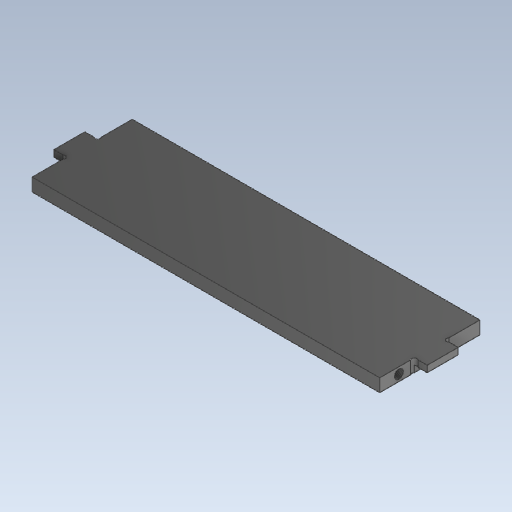
# Autodesk Inventor part: Cockpit_battery_bottom_frame
Saved by Autodesk Inventor 2020 (Build 240168000, 168)
## iProperties
Created: 2022-04-24
Part Number: Cockpit_battery_bottom_frame
Material: アセタール樹脂、黒
Document SubType Name: Modeling
Designer: Masato Kubotera
Density: 1.425 g/cm^3
Appearance: 滑らか - 黒
Description: POM T5
Author: Masato Kubotera
Autodesk Inventor part; units mm, degrees
ref_plane "YZ Plane" through (0, 0, 0) normal (1, 0, 0) x (0, 1, 0)
ref_plane "XZ Plane" through (0, 0, 0) normal (0, 1, 0) x (-1, 0, 0)
derived "Cockpit_side_frame.ipt"
sketch "スケッチ2" plane through (0, 0, 0) normal (0, 1, 0) x (-1, 0, 0)
  line L0 (-23.5, -22.5) -> (-28.5, -27.5)
  line L1 (-28.5, -27.5) -> (-28.5, -91)
  line L2 (-28.5, -91) -> (-23.5, -96)
  line L3 (-23.5, -96) -> (35.75, -96)
  line L4 (37.75, -98) -> (37.75, -131)
  line L5 (37.75, -131) -> (42.75, -136)
  line L6 (42.75, -136) -> (83.5, -136)
  line L7 (88.5, -131) -> (88.5, -20)
  line L8 (88.5, -20) -> (86, -17.5)
  line L9 (86, -17.5) -> (80.25, -17.5)
  line L10 (80.25, -17.5) -> (80.25, -22.5)
  line L11 (80.25, -22.5) -> (73.9849, -22.5)
  line L12 (72.5, -21.0151) -> (72.5, -17.5)
  line L13 (72.5, -17.5) -> (64.5, -17.5)
  line L14 (64.5, -17.5) -> (64.5, -21.0151)
  line L15 (63.0151, -22.5) -> (-23.5, -22.5)
  line L16 (-25.25, -25) -> (-20.25, -25) construction
  line L17 (-20.25, -25) -> (-20.25, -93.5) construction
  line L18 (-20.25, -93.5) -> (-25.25, -93.5) construction
  line L19 (-25.25, -93.5) -> (-25.25, -25) construction
  line L20 (-26, -25) -> (-25.25, -25) construction
  line L21 (-25.25, -93.5) -> (-26, -93.5) construction
  line L22 (-26, -93.5) -> (-26, -25) construction
  line L23 (-20.25, -93.5) -> (80.25, -93.5) construction
  line L24 (-20.25, -88.5) -> (80.25, -88.5) construction
  line L25 (80.25, -22.5) -> (80.25, -90.5) construction
  line L26 (80.25, -90.5) -> (85.25, -90.5) construction
  line L27 (85.25, -90.5) -> (85.25, -22.5) construction
  line L28 (80.25, -88.5) -> (80.25, -93.5) construction
  line L29 (80.25, -91) -> (85.25, -91) construction
  line L30 (85.25, -91) -> (85.25, -133.5) construction
  line L31 (80.25, -91) -> (80.25, -133.5) construction
  line L32 (80.25, -133.5) -> (85.25, -133.5) construction
  line L33 (40.25, -133.5) -> (40.25, -128.5) construction
  line L34 (40.25, -128.5) -> (40.25, -93.5) construction
  line L35 (45.25, -93.5) -> (45.25, -128.5) construction
  line L36 (40.25, -128.5) -> (45.25, -128.5) construction
  line L37 (42.75, -128.5) -> (42.75, -93.5) construction
  line L38 (40.25, -128.5) -> (79.1145, -128.5) construction
  line L39 (79.1145, -128.5) -> (79.1145, -133.5) construction
  line L40 (79.1145, -133.5) -> (40.25, -133.5) construction
  line L41 (40.25, -131) -> (79.1145, -131) construction
  line L42 (82.75, -91) -> (82.75, -133.5) construction
  circle A0 centre (82.75, -131) radius 2
  arc A1 (80.25, -128.5) -> (85.25, -128.5) centre (82.75, -131) ccw construction
  line L43 (80.25, -91) -> (-20.25, -91) construction
  line L44 (42.75, -111) -> (45.25, -111) construction
  line L45 (59.6822, -128.5) -> (59.6822, -131) construction
  line L46 (42.7, -115.5651) -> (42.7, -106.4349)
  line L47 (45.3, -107.05) -> (45.3, -114.95)
  line L48 (45.3, -117.05) -> (42.7, -104.95) construction
  line L49 (42.7, -117.05) -> (45.3, -104.95) construction
  line L50 (55.7322, -128.45) -> (63.6322, -128.45)
  line L51 (64.2473, -131.05) -> (55.1172, -131.05)
  line L52 (53.6322, -128.45) -> (65.7322, -131.05) construction
  line L53 (65.7322, -128.45) -> (53.6322, -131.05) construction
  line L54 (42.75, -105) -> (45.25, -105) construction
  line L55 (42.75, -117) -> (45.25, -117) construction
  arc A2 (44.1849, -104.95) -> (42.7, -106.4349) centre (43.4425, -105.6925) ccw
  arc A3 (45.3, -107.05) -> (45.3, -104.95) centre (45.3, -106) ccw
  arc A4 (42.7, -115.5651) -> (44.1849, -117.05) centre (43.4425, -116.3075) ccw
  arc A5 (45.3, -117.05) -> (45.3, -114.95) centre (45.3, -116) ccw
  line L56 (53.6822, -131) -> (53.6822, -128.5) construction
  line L57 (65.6822, -128.5) -> (65.6822, -131) construction
  arc A6 (53.6322, -129.5651) -> (55.1172, -131.05) centre (54.3747, -130.3075) ccw
  arc A7 (55.7322, -128.45) -> (53.6322, -128.45) centre (54.6822, -128.45) ccw
  arc A8 (64.2473, -131.05) -> (65.7322, -129.5651) centre (64.9898, -130.3075) ccw
  arc A9 (65.7322, -128.45) -> (63.6322, -128.45) centre (64.6822, -128.45) ccw
  line L58 (53.6322, -129.5651) -> (53.6322, -128.45)
  line L59 (65.7322, -128.45) -> (65.7322, -129.5651)
  line L60 (44.1849, -104.95) -> (45.3, -104.95)
  line L61 (45.3, -117.05) -> (44.1849, -117.05)
  circle A10 centre (47.6822, -131) radius 1.6
  line L62 (85.25, -22.5) -> (85.25, -17.5) construction
  line L63 (86, -17.5) -> (86, -90.5) construction
  line L64 (86, -90.5) -> (85.25, -90.5) construction
  line L65 (-18.5, -82.5) -> (-18.5, -61)
  arc A11 (-18.5, -82.5) -> (-16.5, -84.5) centre (-16.5, -82.5) ccw
  line L66 (45.5, -84.5) -> (-16.5, -84.5)
  arc A12 (45.5, -84.5) -> (47.5, -82.5) centre (45.5, -82.5) ccw
  line L67 (47.5, -61) -> (47.5, -82.5)
  arc A13 (47.5, -61) -> (45.5, -59) centre (45.5, -61) ccw
  line L68 (-16.5, -59) -> (45.5, -59)
  arc A14 (-16.5, -59) -> (-18.5, -61) centre (-16.5, -61) ccw
  line L69 (30, -88.5) -> (30, -91) construction
  line L70 (82.75, -22.5) -> (82.75, -90.5) construction
  circle A15 centre (82.75, -34) radius 1.6
  circle A16 centre (82.75, -34) radius 3
  circle A17 centre (82.75, -79) radius 3
  circle A18 centre (82.75, -79) radius 1.6
  line L71 (85.25, -22.5) -> (80.25, -22.5) construction
  arc A19 (85.25, -91) -> (80.25, -91) centre (82.75, -131) ccw construction
  circle A20 centre (47.6822, -131) radius 3
  circle A21 centre (42.75, -99) radius 1.6
  circle A22 centre (42.75, -99) radius 3
  line L72 (5, -88.5) -> (5, -91) construction
  line L73 (55, -88.5) -> (55, -91) construction
  line L74 (53.5651, -91.05) -> (6.4349, -91.05)
  line L75 (4.95, -89.5651) -> (4.95, -88.45)
  line L76 (7.05, -88.45) -> (52.95, -88.45)
  line L77 (55.05, -88.45) -> (55.05, -89.5651)
  line L78 (55.05, -91.05) -> (4.95, -88.45) construction
  line L79 (4.95, -91.05) -> (55.05, -88.45) construction
  arc A23 (7.05, -88.45) -> (4.95, -88.45) centre (6, -88.45) ccw
  arc A24 (4.95, -89.5651) -> (6.4349, -91.05) centre (5.6925, -90.3075) ccw
  arc A25 (53.5651, -91.05) -> (55.05, -89.5651) centre (54.3075, -90.3075) ccw
  arc A26 (55.05, -88.45) -> (52.95, -88.45) centre (54, -88.45) ccw
  line L80 (-20.25, -41) -> (80.25, -41) construction
  line L81 (80.25, -36) -> (-20.25, -36) construction
  line L82 (-20.25, -36) -> (-20.25, -41) construction
  line L83 (-20.25, -38.5) -> (80.25, -38.5) construction
  line L84 (30, -41) -> (30, -36) construction
  line L85 (53.5651, -35.95) -> (6.4349, -35.95)
  line L86 (6.4349, -41.05) -> (53.5651, -41.05)
  line L87 (55.05, -35.95) -> (4.95, -41.05) construction
  line L88 (4.95, -35.95) -> (55.5723, -41.1032) construction
  arc A27 (6.4349, -35.95) -> (4.95, -37.4349) centre (5.6925, -36.6925) ccw
  arc A28 (4.95, -39.5651) -> (6.4349, -41.05) centre (5.6925, -40.3075) ccw
  arc A29 (55.05, -37.4349) -> (53.5651, -35.95) centre (54.3075, -36.6925) ccw
  arc A30 (53.5651, -41.05) -> (55.05, -39.5651) centre (54.3075, -40.3075) ccw
  line L89 (5, -41) -> (5, -36) construction
  line L90 (55, -36) -> (55, -41) construction
  line L91 (4.95, -37.4349) -> (4.95, -39.5651)
  line L92 (55.05, -39.5651) -> (55.05, -37.4349)
  circle A31 centre (-2.5, -38.5) radius 1.6
  circle A32 centre (-2.5, -38.5) radius 3
  circle A33 centre (62.5, -38.5) radius 1.6
  circle A34 centre (62.5, -38.5) radius 3
  line L93 (-25.25, -44.25) -> (-22.75, -44.25) construction
  line L94 (-25.25, -49.25) -> (-26, -49.25) construction
  line L95 (-25.25, -74.25) -> (-22.75, -74.25) construction
  line L96 (-25.25, -69.25) -> (-26, -69.25) construction
  line L97 (-26, -59.25) -> (-25.25, -59.25) construction
  line L98 (-25.25, -59.25) -> (-22.75, -59.25) construction
  line L99 (-22.75, -25) -> (-22.75, -93.5) construction
  arc A35 (63.0151, -22.5) -> (64.5, -21.0151) centre (63.7575, -21.7575) ccw
  arc A36 (72.5, -21.0151) -> (73.9849, -22.5) centre (73.2425, -21.7575) ccw
  line L100 (56.75, -22.5) -> (56.75, -32.5) construction
  line L101 (56.75, -32.5) -> (80.25, -32.5) construction
  line L102 (80.25, -32.5) -> (80.25, -22.5) construction
  line L103 (68.5, -17.5) -> (68.5, -32.5) construction
  line L104 (60.5, -22.5) -> (60.5, -17.5) construction
  line L105 (76.5, -22.5) -> (76.5, -17.5) construction
  line L106 (-22.7, -46.3) -> (-22.7, -72.2)
  line L107 (-25.3, -72.8151) -> (-25.3, -69.564)
  line L108 (-25.3, -44.2) -> (-22.7, -74.3) construction
  line L109 (-22.7, -44.2) -> (-25.3, -74.3) construction
  arc A37 (-22.7, -46.3) -> (-22.7, -44.2) centre (-22.7, -45.25) ccw
  arc A38 (-23.8151, -44.2) -> (-25.3, -45.6849) centre (-24.5575, -44.9425) ccw
  line L110 (-23.8151, -44.2) -> (-22.7, -44.2)
  arc A39 (-25.3, -72.8151) -> (-23.8151, -74.3) centre (-24.5575, -73.5575) ccw
  arc A40 (-22.7, -74.3) -> (-22.7, -72.2) centre (-22.7, -73.25) ccw
  line L111 (-22.7, -74.3) -> (-23.8151, -74.3)
  line L112 (-26.3, -49.9848) -> (-26.3, -68.5152)
  arc A41 (-26.3, -68.5152) -> (-25.3, -69.564) centre (-25.25, -68.5152) ccw
  arc A42 (-25.3, -48.936) -> (-26.3, -49.9848) centre (-25.25, -49.9848) ccw
  line L113 (-25.3, -48.936) -> (-25.3, -45.6849)
  circle A43 centre (-22.75, -36.75) radius 1.6
  circle A44 centre (-22.75, -36.75) radius 3
  circle A45 centre (-22.75, -81.75) radius 1.6
  circle A46 centre (-22.75, -81.75) radius 3
  line L114 (64.5, -22.5) -> (72.5, -22.5)
  line L115 (85.25, -17.5) -> (52.5, -17.5) construction
  line L116 (52.5, -17.5) -> (52.5, -22.5) construction
  circle A47 centre (82.75, -93.5) radius 1.475
  circle A48 centre (82.75, -98.5) radius 1.475
  circle A49 centre (82.75, -103.5) radius 1.475
  line L117 (49.75, -93.5) -> (78.25, -93.5)
  line L118 (80.25, -95.5) -> (80.25, -124)
  line L119 (78.25, -126) -> (49.75, -126)
  line L120 (47.75, -124) -> (47.75, -95.5)
  arc A50 (49.75, -93.5) -> (47.75, -95.5) centre (49.75, -95.5) ccw
  arc A51 (47.75, -124) -> (49.75, -126) centre (49.75, -124) ccw
  arc A52 (78.25, -126) -> (80.25, -124) centre (78.25, -124) ccw
  arc A53 (80.25, -95.5) -> (78.25, -93.5) centre (78.25, -95.5) ccw
  arc A54 (37.75, -98) -> (35.75, -96) centre (35.75, -98) ccw
  circle A55 centre (-13.5, -55) radius 1.75
  circle A56 centre (-13.5, -55) radius 2
  line L121 (74.85, -78.65) -> (65.65, -78.65) construction
  line L122 (65.65, -78.65) -> (65.65, -64.85) construction
  line L123 (65.65, -64.85) -> (74.85, -64.85) construction
  line L124 (74.85, -64.85) -> (74.85, -78.65) construction
  line L125 (74.85, -78.65) -> (65.65, -64.85) construction
  line L126 (65.65, -78.65) -> (74.85, -64.85) construction
  line L127 (64.95, -64.2) -> (75.55, -64.2) construction
  line L128 (75.55, -64.2) -> (75.55, -79.3) construction
  line L129 (75.55, -79.3) -> (64.95, -79.3) construction
  line L130 (64.95, -79.3) -> (64.95, -64.2) construction
  line L131 (64.95, -64.2) -> (75.55, -79.3) construction
  line L132 (75.55, -64.2) -> (64.95, -79.3) construction
  line L133 (66.3849, -64.15) -> (74.1151, -64.15)
  line L134 (75.6, -65.6349) -> (75.6, -77.8651)
  line L135 (75.6, -79.35) -> (64.9, -64.15) construction
  line L136 (64.9, -79.35) -> (75.6, -64.15) construction
  line L137 (74.9, -78.7) -> (65.6, -64.8) construction
  line L138 (65.6, -78.7) -> (74.9, -64.8) construction
  arc A57 (66.3849, -64.15) -> (64.9, -65.6349) centre (65.6425, -64.8925) ccw
  arc A58 (67.0849, -64.8) -> (65.6, -66.2849) centre (66.3425, -65.5425) ccw
  line L139 (64.9, -71.75) -> (75.6, -71.75) construction
  line L140 (70.25, -64.15) -> (70.25, -78.7063) construction
  arc A59 (75.6, -65.6349) -> (74.1151, -64.15) centre (74.8575, -64.8925) ccw
  arc A60 (74.9, -66.2849) -> (73.4151, -64.8) centre (74.1575, -65.5425) ccw
  arc A61 (65.6, -77.2151) -> (67.0849, -78.7) centre (66.3425, -77.9575) ccw
  arc A62 (64.9, -77.8651) -> (66.3849, -79.35) centre (65.6425, -78.6075) ccw
  arc A63 (73.4151, -78.7) -> (74.9, -77.2151) centre (74.1575, -77.9575) ccw
  arc A64 (74.1151, -79.35) -> (75.6, -77.8651) centre (74.8575, -78.6075) ccw
  line L141 (67.0849, -64.8) -> (73.4151, -64.8)
  line L142 (74.9, -66.2849) -> (74.9, -77.2151)
  line L143 (64.9, -77.8651) -> (64.9, -65.6349)
  line L144 (65.6, -77.2151) -> (65.6, -66.2849)
  line L145 (73.4151, -78.7) -> (67.0849, -78.7)
  line L146 (74.1151, -79.35) -> (66.3849, -79.35)
  line L147 (-18.5, -71.75) -> (47.5, -71.75) construction
  line L148 (82.75, -56.5) -> (85.25, -56.5) construction
  line L149 (86, -54) -> (85.25, -54) construction
  line L150 (82.7, -69.45) -> (82.7, -43.55)
  line L151 (85.3057, -71.616) -> (82.7, -41.45) construction
  line L152 (82.7, -71.55) -> (85.3, -41.45) construction
  arc A65 (82.7, -41.45) -> (82.7, -43.55) centre (82.7, -42.5) ccw
  arc A66 (85.3, -42.9349) -> (83.8151, -41.45) centre (84.5575, -42.1925) ccw
  arc A67 (82.7, -69.45) -> (82.7, -71.55) centre (82.7, -70.5) ccw
  arc A68 (83.8151, -71.55) -> (85.3, -70.0651) centre (84.5575, -70.8075) ccw
  line L153 (82.75, -41.5) -> (85.25, -41.5) construction
  line L154 (82.75, -71.5) -> (85.25, -71.5) construction
  arc A69 (86.25, -47.1801) -> (85.3, -46.1348) centre (85.2, -47.1801) ccw
  line L155 (86.25, -47.1801) -> (86.25, -65.8199)
  line L156 (85.25, -46.5) -> (86, -46.5) construction
  line L157 (85.25, -66.5) -> (86, -66.5) construction
  arc A70 (85.3, -66.8652) -> (86.25, -65.8199) centre (85.2, -65.8199) ccw
  line L158 (85.3, -42.9349) -> (85.3, -46.1348)
  line L159 (85.3, -66.8652) -> (85.3, -70.0651)
  line L160 (83.8151, -71.55) -> (82.7, -71.55)
  line L161 (82.7, -41.45) -> (83.8151, -41.45)
  line L162 (83.5, -136) -> (88.5, -131)
  point P0 (0, 0)
  point P1 (-25.7227, -96)
  point P2 (-23.5, -22.5)
  point P3 (44, -111)
  point P4 (59.6822, -129.75)
  point P5 (30, -89.75)
  point P6 (30, -38.5)
  point P7 (4.95, -41.05)
  point P8 (52.5, -22)
  point P9 (-24, -59.25)
  point P10 (70.25, -71.75)
  point P11 (70.25, -71.75)
  point P12 (84, -56.5)
  dimension "d1" = 128.5
  dimension "d2" = 5
  dimension "d3" = 2.5
  measures "d1" vertical distance of L33.end point (0, 0)
  measures "d2" distance of L33.start L33.end
  measures "d3" distance of L56.start L56.end
ref_plane "作業平面1" through (0, 0, -128.5) normal (0, 0, 1) x (1, 0, 0)
sketch "スケッチ3" plane through (0, 0, -128.5) normal (0, 0, 1) x (1, 0, 0)
  line L0 (-40.25, -135) -> (-40.25, 0)
  line L1 (-79.1145, 0) -> (-79.1145, -135)
  line L2 (-65.6822, 1.4849) -> (-65.6822, 5)
  line L3 (-65.6822, 5) -> (-53.6822, 5)
  line L4 (-59.6822, -135) -> (-59.6822, 0) construction
  line L5 (-79.1145, -67.5) -> (-40.25, -67.5) construction
  arc A0 (-67.1672, 0) -> (-65.6822, 1.4849) centre (-66.4247, 0.7425) ccw
  line L6 (-67.1672, 0) -> (-79.1145, 0)
  line L7 (-53.6822, 1.4849) -> (-53.6822, 5)
  arc A1 (-53.6822, 1.4849) -> (-52.1973, 0) centre (-52.9398, 0.7425) ccw
  line L8 (-52.1973, 0) -> (-40.25, 0)
  line L9 (-40.25, 0) -> (-52.1973, 0)
  line L10 (-53.6822, 0) -> (-65.6822, 0)
  line L11 (-65.6822, -136.4849) -> (-65.6822, -140)
  line L12 (-65.6822, -140) -> (-53.6822, -140)
  arc A2 (-65.6822, -136.4849) -> (-67.1672, -135) centre (-66.4247, -135.7425) ccw
  line L13 (-67.1672, -135) -> (-79.1145, -135)
  line L14 (-52.1973, -135) -> (-40.25, -135)
  arc A3 (-52.1973, -135) -> (-53.6822, -136.4849) centre (-52.9398, -135.7425) ccw
  line L15 (-53.6822, -136.4849) -> (-53.6822, -140)
  line L16 (-53.6822, -135) -> (-65.6822, -135)
  line L17 (-50.6145, -14) -> (-44.75, -14)
  line L18 (-42.75, -12) -> (-42.75, -6)
  line L19 (-44.75, -4) -> (-50.6145, -4)
  line L20 (-52.6145, -6) -> (-52.6145, -12)
  line L21 (-42.75, -116.5) -> (-42.75, -18.5)
  line L22 (-44.75, -16.5) -> (-50.8824, -16.5)
  line L23 (-52.8747, -18.3252) -> (-57.1746, -67.3252)
  line L24 (-57.6899, -44.5988) -> (-55.1221, -15.3372)
  line L25 (-55.1145, -15.1624) -> (-55.1145, -6)
  line L26 (-57.1145, -4) -> (-62.25, -4)
  line L27 (-68.75, -14) -> (-74.6145, -14)
  line L28 (-76.6145, -12) -> (-76.6145, -6)
  line L29 (-74.6145, -4) -> (-68.75, -4)
  line L30 (-66.75, -6) -> (-66.75, -12)
  line L31 (-76.6145, -116.5) -> (-76.6145, -18.5)
  line L32 (-74.6145, -16.5) -> (-68.4821, -16.5)
  line L33 (-66.4898, -18.3252) -> (-62.1899, -67.3252)
  line L34 (-61.6746, -44.5988) -> (-64.2423, -15.3372)
  line L35 (-64.25, -15.1624) -> (-64.25, -6)
  line L36 (-44.75, -118.5) -> (-50.8824, -118.5)
  line L37 (-52.8747, -116.6748) -> (-57.1746, -67.6748)
  line L38 (-66.4898, -116.6748) -> (-62.1899, -67.6748)
  line L39 (-74.6145, -118.5) -> (-68.4821, -118.5)
  line L40 (-47.6822, -4) -> (-47.6822, 0) construction
  arc A4 (-44.75, -118.5) -> (-42.75, -116.5) centre (-44.75, -116.5) ccw
  arc A5 (-52.8747, -116.6748) -> (-50.8824, -118.5) centre (-50.8824, -116.5) ccw
  arc A6 (-68.4821, -118.5) -> (-66.4898, -116.6748) centre (-68.4821, -116.5) ccw
  arc A7 (-76.6145, -116.5) -> (-74.6145, -118.5) centre (-74.6145, -116.5) ccw
  arc A8 (-62.1899, -67.6748) -> (-62.1899, -67.3252) centre (-64.1822, -67.5) ccw
  arc A9 (-57.1746, -67.3252) -> (-57.1746, -67.6748) centre (-55.1822, -67.5) ccw
  arc A10 (-61.6746, -44.5988) -> (-57.6899, -44.5988) centre (-59.6822, -44.4239) ccw
  arc A11 (-66.4898, -18.3252) -> (-68.4821, -16.5) centre (-68.4821, -18.5) ccw
  arc A12 (-74.6145, -16.5) -> (-76.6145, -18.5) centre (-74.6145, -18.5) ccw
  arc A13 (-50.8824, -16.5) -> (-52.8747, -18.3252) centre (-50.8824, -18.5) ccw
  arc A14 (-42.75, -18.5) -> (-44.75, -16.5) centre (-44.75, -18.5) ccw
  arc A15 (-44.75, -14) -> (-42.75, -12) centre (-44.75, -12) ccw
  arc A16 (-42.75, -6) -> (-44.75, -4) centre (-44.75, -6) ccw
  arc A17 (-50.6145, -4) -> (-52.6145, -6) centre (-50.6145, -6) ccw
  arc A18 (-52.6145, -12) -> (-50.6145, -14) centre (-50.6145, -12) ccw
  arc A19 (-55.1221, -15.3372) -> (-55.1145, -15.1624) centre (-57.1145, -15.1624) ccw
  arc A20 (-55.1145, -6) -> (-57.1145, -4) centre (-57.1145, -6) ccw
  arc A21 (-62.25, -4) -> (-64.25, -6) centre (-62.25, -6) ccw
  arc A22 (-64.25, -15.1624) -> (-64.2423, -15.3372) centre (-62.25, -15.1624) ccw
  arc A23 (-68.75, -14) -> (-66.75, -12) centre (-68.75, -12) ccw
  arc A24 (-66.75, -6) -> (-68.75, -4) centre (-68.75, -6) ccw
  arc A25 (-76.6145, -12) -> (-74.6145, -14) centre (-74.6145, -12) ccw
  arc A26 (-74.6145, -4) -> (-76.6145, -6) centre (-74.6145, -6) ccw
  line L41 (-50.6145, -121) -> (-44.75, -121)
  line L42 (-44.75, -131) -> (-50.6145, -131)
  line L43 (-52.6145, -129) -> (-52.6145, -123)
  line L44 (-57.6899, -90.4012) -> (-55.1221, -119.6628)
  line L45 (-55.1145, -119.8376) -> (-55.1145, -129)
  line L46 (-61.6746, -90.4012) -> (-64.2423, -119.6628)
  line L47 (-64.25, -119.8376) -> (-64.25, -129)
  line L48 (-68.75, -121) -> (-74.6145, -121)
  line L49 (-66.75, -129) -> (-66.75, -123)
  line L50 (-76.6145, -123) -> (-76.6145, -129)
  line L51 (-74.6145, -131) -> (-68.75, -131)
  arc A27 (-57.6899, -90.4012) -> (-61.6746, -90.4012) centre (-59.6822, -90.5761) ccw
  arc A28 (-42.75, -123) -> (-44.75, -121) centre (-44.75, -123) ccw
  arc A29 (-44.75, -131) -> (-42.75, -129) centre (-44.75, -129) ccw
  arc A30 (-52.6145, -129) -> (-50.6145, -131) centre (-50.6145, -129) ccw
  arc A31 (-50.6145, -121) -> (-52.6145, -123) centre (-50.6145, -123) ccw
  arc A32 (-55.1145, -119.8376) -> (-55.1221, -119.6628) centre (-57.1145, -119.8376) ccw
  arc A33 (-57.1145, -131) -> (-55.1145, -129) centre (-57.1145, -129) ccw
  arc A34 (-64.25, -129) -> (-62.25, -131) centre (-62.25, -129) ccw
  arc A35 (-64.2423, -119.6628) -> (-64.25, -119.8376) centre (-62.25, -119.8376) ccw
  arc A36 (-66.75, -123) -> (-68.75, -121) centre (-68.75, -123) ccw
  arc A37 (-68.75, -131) -> (-66.75, -129) centre (-68.75, -129) ccw
  arc A38 (-74.6145, -121) -> (-76.6145, -123) centre (-74.6145, -123) ccw
  arc A39 (-76.6145, -129) -> (-74.6145, -131) centre (-74.6145, -129) ccw
  line L52 (-42.75, -123) -> (-42.75, -129)
  line L53 (-57.1145, -131) -> (-62.25, -131)
  point P0 (0, 0)
  point P1 (-65.6822, 0)
  point P2 (-53.6822, 0)
  point P3 (-40.25, 0)
  point P4 (-59.6822, -67.5)
  point P5 (-52.6145, -14)
  point P6 (-42.75, -4)
  point P7 (-42.75, -14)
  point P8 (-52.6145, -4)
  point P9 (-42.75, -118.5)
  point P10 (-42.75, -16.5)
  point P11 (-52.7145, -16.5)
  point P12 (-57.1899, -67.5)
  point P13 (-59.6822, -67.3029)
  point P14 (-55.1145, -15.25)
  point P15 (-55.1145, -4)
  point P16 (-66.75, -14)
  point P17 (-76.6145, -4)
  point P18 (-76.6145, -14)
  point P19 (-66.75, -4)
  point P20 (-76.6145, -16.5)
  point P21 (-66.6499, -16.5)
  point P22 (-62.1745, -67.5)
  point P23 (-64.25, -15.25)
  point P24 (-64.25, -4)
  point P25 (-42.75, -118.5)
  point P26 (-52.7145, -118.5)
  point P27 (-66.6499, -118.5)
  point P28 (-76.6145, -118.5)
  dimension "d5" = 135
  dimension "d7" = 1.05
  dimension "d8" = 5
  dimension "d20" = 4
  dimension "d21" = 2.5
  dimension "d22" = 2.5
  dimension "d23" = 10
  dimension "d24" = 11.25
  dimension "d25" = 2.5
  dimension "d26" = 2.5
  dimension "d27" = 2
  dimension "d28" = 5
  constraints: 108 end point, 83 point on circle, 67 symmetric about line, 54 point on line, 46 tangent, 40 centre point, 22 equal radius, 7 perpendicular, 6 midpoint, 4 parallel, 3 collinear, 2 coincident, 2 vertical, 1 horizontal, 16 other
  measures "d5" distance of L1.start L1.end
  measures "d7" radius of A0
  measures "d8" distance between parallel lines of L3 L10
  measures "d20" distance between parallel lines of L8 L19
  measures "d21" distance between parallel lines of L0 L18
  measures "d22" distance between parallel lines of L22 L17
  measures "d23" distance of point (-42.75, -14) point (-42.75, -4)
  measures "d24" distance of point (-55.114, -15.25) point (-55.114, -4)
  measures "d25" distance between parallel lines of L23 L24
  measures "d26" distance between parallel lines of L20 L25
  measures "d27" radius of A4
extrude "押し出し1" add sketch "スケッチ3" against normal blind 5 contours L14 A3 L16 A2 L13 L1 L6 A0 L10 A1 L8 L0
extrude "押し出し2" add sketch "スケッチ3" against normal blind 2.5 contours A3 L15 L12 L11 A2 L16 | L10 A0 L2 L3 L7 A1
hole "穴1" at (-47.6822, 0, -131) direction (0, -1, 0) diameter 3.4587 depth 4 thread size "M4x0.5" class "6H" standard "ANSI Metric M Profile"
ref_plane "作業平面2" through (-40.25, -67.5, -128.5) normal (0, 1, 0) x (1, 0, 0)
mirror "ミラー1" about plane through (-40.25, -67.5, -128.5) normal (0, 1, 0) of "穴1"
extrude "押し出し3" add sketch "スケッチ3" against normal blind 0.5 contours A18 L20 A17 L19 A16 L18 A15 L17 | A4 L36 A5 L37 A9 L23 A13 L22 A14 L21 | A10 L34 A22 L35 A21 L26 A20 L25 A19 L24 | L27 A25 L28 A26 L29 A24 L30 A23 | L31 A12 L32 A11 L33 A8 L38 A6 L39 A7 | L41 A28 L52 A29 L42 A30 L43 A31 | L44 A32 L45 A33 L53 A34 L47 A35 L46 A27 | A36 L49 A37 L51 A39 L50 A38 L48
equation "\"d22\" = d21"
equation "\"d24\" = d23 + 0.5 * d22"
equation "\"d25\" = d21"
equation "\"d26\" = d21"
equation "\"d28\" = 2 * d21"
equation "\"d9\" = d2"
equation "\"d11\" = d3"
equation "\"d4\" = -d1"
